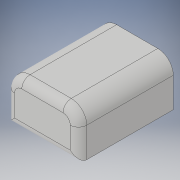
# Autodesk Inventor part: Aquamote3.2_housing_body_version2
Saved by Autodesk Inventor 2019 (Build 230136000, 136)
## iProperties
Created: 2018-04-22
Part Number: Aquamote3.2_housing_body_version2
Material: Generic
Document SubType Name: Modeling
Designer: Leon
Density: 1 g/cm^3
Appearance: Default
Author: Leon
Autodesk Inventor part; units mm, degrees
ref_plane "YZ Plane" through (0, 0, 0) normal (1, 0, 0) x (0, 1, 0)
ref_plane "XZ Plane" through (0, 0, 0) normal (0, 1, 0) x (-1, 0, 0)
ref_plane "XY Plane" through (0, 0, 0) normal (0, 0, 1) x (1, 0, 0)
sketch "Sketch1" plane through (0, 0, 0) normal (0, 0, 1) x (1, 0, 0)
  line L0 (0, 0) -> (35, 0)
  line L1 (35, 0) -> (35, 14.5)
  line L2 (27.5, 22) -> (7.5, 22)
  line L3 (0, 14.5) -> (0, 0)
  arc A0 (7.5, 22) -> (0, 14.5) centre (7.5, 14.5) ccw
  arc A1 (35, 14.5) -> (27.5, 22) centre (27.5, 14.5) ccw
  point P0 (35, 22)
  point P1 (0, 22)
  dimension "d0" = 35
  dimension "d1" = 22
  dimension "d2" = 7.5
  constraints: 8 end point, 4 point on circle, 4 point on line, 4 tangent, 2 centre point, 2 parallel, 1 equal radius, 1 horizontal, 1 perpendicular
  measures "d0" distance of point (0, 22) point (35, 22)
  measures "d1" distance of point (35, 22) L0.end
  measures "d2" radius of A0
extrude "Extrusion1" add sketch "Sketch1" along normal blind 46
sketch "Sketch2" plane through (0, 0, 0) normal (0, 0, -1) x (-1, 0, 0)
  line L0 (-9.5, 3) -> (-25.5, 3)
  line L1 (-29, 6.5) -> (-29, 15.5)
  line L2 (-25.5, 19) -> (-9.5, 19)
  line L3 (-6, 15.5) -> (-6, 14.8)
  arc A0 (-25.5, 19) -> (-29, 15.5) centre (-25.5, 15.5) ccw
  arc A1 (-29, 6.5) -> (-25.5, 3) centre (-25.5, 6.5) ccw
  arc A2 (-9.5, 3) -> (-6, 6.5) centre (-9.5, 6.5) ccw
  arc A3 (-6, 15.5) -> (-9.5, 19) centre (-9.5, 15.5) ccw
  line L4 (-29, 14.8) -> (-30.3, 14.8)
  line L5 (-30.3, 14.8) -> (-30.3, 13.2)
  line L6 (-30.3, 13.2) -> (-29, 13.2)
  line L7 (-29, 13.2) -> (-29, 14.8)
  line L8 (-6, 14.8) -> (-6, 13.2)
  line L9 (-6, 13.2) -> (-6, 6.5)
  line L10 (-6, 6.5) -> (-6, 15.5)
  line L11 (-6, 14.8) -> (-4.7, 14.8)
  line L12 (-4.7, 14.8) -> (-4.7, 13.2)
  line L13 (-4.7, 13.2) -> (-6, 13.2)
  point P0 (0, 0)
  point P1 (-29, 19)
  point P2 (-29, 3)
  point P3 (-6, 19)
  dimension "d5" = 23
  dimension "d6" = 16
  dimension "d7" = 3.5
  dimension "d8" = 6
  dimension "d9" = 19
  dimension "d80" = 1.3
  dimension "d81" = 1.6
  dimension "d82" = 4.2
  dimension "d88" = 1.3
  dimension "d89" = 1.6
  dimension "d90" = 4.2
  constraints: 28 end point, 13 tangent, 9 parallel, 8 point on circle, 6 point on line, 4 centre point, 3 equal radius, 2 horizontal, 2 perpendicular
  measures "d5" distance of point (-29, 19) point (-6, 19)
  measures "d6" distance of point (-29, 3) point (-29, 19)
  measures "d7" radius of A0
  measures "d8" distance from line of point (0, 0) L3
  measures "d9" distance from line of point (0, 0) L2
  measures "d80" distance of L6.end L5.end
  measures "d81" distance of L5.end L4.end
  measures "d82" distance between parallel lines of L2 L4
  measures "d88" distance between parallel lines of L12 L3
  measures "d89" distance between parallel lines of L11 L13
  measures "d90" distance between parallel lines of L11 L2
extrude "Extrusion2" cut sketch "Sketch2" against normal blind 43 contours L0 A1 L1 A0 L2 A3 L3 L8 L9 A2
chamfer "Chamfer1" distance 2 distance2 2.2 7 edges at (29, 11, 0) (27.9749, 17.9749, 0) (17.5, 19, 0) (7.0251, 17.9749, 0) (7.0251, 4.0251, 0) (17.5, 3, 0) (27.9749, 4.0251, 0) measured on face at (14.8333, 1, 0)
fillet "Fillet1" radius 2 7 edges at (29, 11, 43) (27.9749, 4.0251, 43) (17.5, 3, 43) (7.0251, 4.0251, 43) (7.0251, 17.9749, 43) (17.5, 19, 43) (27.9749, 17.9749, 43)
fillet "Fillet2" radius 4 6 edges at (17.5, 0, 46) (35, 7.25, 46) (32.8033, 19.8033, 46) (17.5, 22, 46) (2.1967, 19.8033, 46) (0, 7.25, 46)
sketch "Sketch4" plane through (0, 0, 0) normal (0, 0, -1) x (-1, 0, 0)
  circle A0 centre (-2, 11) radius 1.5
  line L0 (0, 14.5) -> (0, 0) projected
  line L1 (0, 0) -> (-35, 0) projected
  circle A1 centre (-33, 11) radius 1.5
  dimension "d20" = 3
  dimension "d21" = 2
  dimension "d22" = 11
  dimension "d23" = 3
  dimension "d24" = 11
  dimension "d25" = 31
  constraints: 2 centre point
  measures "d20" diameter of A0
  measures "d21" distance from line of L0 A0.centre
  measures "d22" distance from line of L1 A0.centre
  measures "d23" diameter of A1
  measures "d24" distance from line of L1 A1.centre
  measures "d25" distance of A0.centre A1.centre
hole "Hole1" at (2, 11, 0) direction (0, 0, 1) diameter 3 depth 15 tip angle 118
hole "Hole2" at (33, 11, 0) direction (0, 0, 1) diameter 3 depth 15 tip angle 118
thread "Thread1" size "M3x0.5" class "6H" standard "ANSI Metric M Profile" full length
thread "Thread2" size "M3x0.5" class "6H" standard "ANSI Metric M Profile" full length
sketch "Sketch6" plane through (33, 11, 0) normal (1, 0, 0) x (0, 1, 0)
  line L0 (1.5, 0) -> (1.5, 15)
  line L1 (1.5, 15) -> (1.1293, 15)
  line L2 (1.1293, 15) -> (1.1293, 0)
  line L3 (1.1293, 0) -> (1.5, 0)
  line L4 (0, -3) -> (0, 18) projected
  constraints: 8 end point
revolve "Revolution1" add sketch "Sketch6" angle 360 about axis through (33, 11, 0) along (0, 0, 1) separate body
sketch "Sketch5" plane through (33, 12.5, 0) normal (-1, 0, 0) x (0, 0, 1)
  line L0 (-0.2918, -0.0255) -> (-0.2501, -0.0255) construction
  line L1 (0.0416, -0.3456) -> (-0.0001, -0.4257) construction
  line L2 (-0.5001, -0.4257) -> (-0.5418, -0.3456) construction
  line L3 (-0.2084, -0.0255) -> (-0.2501, 0.0546) construction
  line L4 (-0.2501, 0.0546) -> (-0.2918, -0.0255) construction
  line L5 (-0.5001, -0.4257) -> (-0.4584, -0.3456) construction
  line L6 (-0.2084, -0.0255) -> (-0.0418, -0.3456)
  line L7 (-0.5418, -0.3456) -> (-0.4584, -0.3456) construction
  arc A0 (-0.5418, -0.3456) -> (-0.5001, -0.3709) centre (-0.5001, -0.3239) ccw construction
  line L8 (0.0416, -0.3456) -> (-0.0418, -0.3456) construction
  line L9 (-0.5001, -0.4257) -> (-0.5001, -0.3456) construction
  line L10 (-0.0001, -0.4257) -> (-0.0001, -0.3456) construction
  line L11 (-0.2501, 0.0546) -> (-0.2501, -0.0002) construction
  line L12 (-0.5001, -0.3709) -> (-0.0001, -0.3709)
  arc A1 (-0.5001, -0.3709) -> (-0.4584, -0.3456) centre (-0.5001, -0.3239) ccw
  line L13 (-0.0418, -0.3456) -> (-0.0001, -0.4257) construction
  line L14 (-0.4584, -0.3456) -> (-0.2918, -0.0255)
  line L15 (-0.0001, -0.0002) -> (-0.0001, 0.0177)
  line L16 (-0.0001, 0.0177) -> (-0.0001, -0.0002)
  line L17 (-0.0001, -0.0002) -> (0.0334, -0.0002)
  arc A2 (-0.0418, -0.3456) -> (-0.0001, -0.3709) centre (-0.0001, -0.3239) ccw
  arc A3 (-0.0001, -0.3709) -> (0.0416, -0.3456) centre (-0.0001, -0.3239) ccw construction
  arc A4 (-0.2501, -0.0002) -> (-0.2918, -0.0255) centre (-0.2501, -0.0471) ccw
  arc A5 (-0.2084, -0.0255) -> (-0.2501, -0.0002) centre (-0.2501, -0.0471) ccw
  line L18 (-0.2501, -0.0002) -> (-0.2501, -0.0255) construction
  line L19 (-0.2501, -0.0255) -> (-0.2084, -0.0255) construction
  dimension "d44" = 55
  dimension "d45" = 0.08
  dimension "d46" = 0.08
  dimension "Sketch5_ThreadOffset" = 0
  dimension "Sketch5_MajorRadius" = 0.3707
  dimension "d49" = 0.5
  dimension "Sketch5_MinorRadius" = 0
  constraints: 40 end point, 12 point on circle, 10 parallel, 8 tangent, 6 centre point, 6 collinear, 2 midpoint, 2 point on line, 1 horizontal, 1 perpendicular, 3 other
  measures "d44" angle of L6 L14
  measures "d45" distance of L3.end L0.end
  measures "d46" distance of L1.end L10.end
  measures "Sketch5_ThreadOffset" distance between parallel lines of L15 L10
  measures "Sketch5_MajorRadius" distance from line of L12 L15.start
  measures "d49" distance from line of L1.end L9
  measures "Sketch5_MinorRadius" distance edge to line of A5 L17
coil "Coil1" sketch "Sketch5" operation cut axis through (33, 11, 0) along (0, 0, 1) pitch 0.5005 turns 31.968032 hand right bodies 2
sketch "Sketch8" plane through (2, 11, 0) normal (1, 0, 0) x (0, 1, 0)
  line L0 (1.5, 0) -> (1.5, 15)
  line L1 (1.5, 15) -> (1.1293, 15)
  line L2 (1.1293, 15) -> (1.1293, 0)
  line L3 (1.1293, 0) -> (1.5, 0)
  line L4 (0, -3) -> (0, 18) projected
  constraints: 8 end point
revolve "Revolution2" add sketch "Sketch8" angle 360 about axis through (2, 11, 0) along (0, 0, 1) separate body
sketch "Sketch7" plane through (2, 12.5, 0) normal (-1, 0, 0) x (0, 0, 1)
  line L0 (-0.2918, -0.0255) -> (-0.2501, -0.0255) construction
  line L1 (0.0416, -0.3456) -> (-0.0001, -0.4257) construction
  line L2 (-0.5001, -0.4257) -> (-0.5418, -0.3456) construction
  line L3 (-0.2084, -0.0255) -> (-0.2501, 0.0546) construction
  line L4 (-0.2501, 0.0546) -> (-0.2918, -0.0255) construction
  line L5 (-0.5001, -0.4257) -> (-0.4584, -0.3456) construction
  line L6 (-0.2084, -0.0255) -> (-0.0418, -0.3456)
  line L7 (-0.5418, -0.3456) -> (-0.4584, -0.3456) construction
  arc A0 (-0.5418, -0.3456) -> (-0.5001, -0.3709) centre (-0.5001, -0.3239) ccw construction
  line L8 (0.0416, -0.3456) -> (-0.0418, -0.3456) construction
  line L9 (-0.5001, -0.4257) -> (-0.5001, -0.3456) construction
  line L10 (-0.0001, -0.4257) -> (-0.0001, -0.3456) construction
  line L11 (-0.2501, 0.0546) -> (-0.2501, -0.0002) construction
  line L12 (-0.5001, -0.3709) -> (-0.0001, -0.3709)
  arc A1 (-0.5001, -0.3709) -> (-0.4584, -0.3456) centre (-0.5001, -0.3239) ccw
  line L13 (-0.0418, -0.3456) -> (-0.0001, -0.4257) construction
  line L14 (-0.4584, -0.3456) -> (-0.2918, -0.0255)
  line L15 (-0.0001, -0.0002) -> (-0.0001, 0.0177)
  line L16 (-0.0001, 0.0177) -> (-0.0001, -0.0002)
  line L17 (-0.0001, -0.0002) -> (0.0334, -0.0002)
  arc A2 (-0.0418, -0.3456) -> (-0.0001, -0.3709) centre (-0.0001, -0.3239) ccw
  arc A3 (-0.0001, -0.3709) -> (0.0416, -0.3456) centre (-0.0001, -0.3239) ccw construction
  arc A4 (-0.2501, -0.0002) -> (-0.2918, -0.0255) centre (-0.2501, -0.0471) ccw
  arc A5 (-0.2084, -0.0255) -> (-0.2501, -0.0002) centre (-0.2501, -0.0471) ccw
  line L18 (-0.2501, -0.0002) -> (-0.2501, -0.0255) construction
  line L19 (-0.2501, -0.0255) -> (-0.2084, -0.0255) construction
  dimension "d62" = 55
  dimension "d63" = 0.08
  dimension "d64" = 0.08
  dimension "Sketch7_ThreadOffset" = 0
  dimension "Sketch7_MajorRadius" = 0.3707
  dimension "d67" = 0.5
  dimension "Sketch7_MinorRadius" = 0
  constraints: 40 end point, 12 point on circle, 10 parallel, 8 tangent, 6 centre point, 6 collinear, 2 midpoint, 2 point on line, 1 horizontal, 1 perpendicular, 3 other
  measures "d62" angle of L6 L14
  measures "d63" distance of L3.end L0.end
  measures "d64" distance of L1.end L10.end
  measures "Sketch7_ThreadOffset" distance between parallel lines of L15 L10
  measures "Sketch7_MajorRadius" distance from line of L12 L15.start
  measures "d67" distance from line of L1.end L9
  measures "Sketch7_MinorRadius" distance edge to line of A5 L17
coil "Coil2" sketch "Sketch7" operation cut axis through (2, 11, 0) along (0, 0, 1) pitch 0.5005 turns 31.968032 hand right bodies 3
extrude "Extrusion3" cut sketch "Sketch2" against normal blind 42 contours L6 L5 L4 L1 bodies 1
extrude "Extrusion4" cut sketch "Sketch2" against normal blind 42 contours L8 L11 L12 L13 bodies 1
equation "\"d44\" = d51"
equation "\"d45\" = 0.160083 * Sketch5_Pitch"
equation "\"d46\" = 0.160083 * Sketch5_Pitch"
equation "\"d49\" = Sketch5_Pitch"
equation "\"d62\" = d69"
equation "\"d63\" = 0.160083 * Sketch7_Pitch"
equation "\"d64\" = 0.160083 * Sketch7_Pitch"
equation "\"d67\" = Sketch7_Pitch"
equation "\"d51\" = 55deg"
equation "\"Sketch5_Pitch\" = 0.5"
equation "\"d69\" = 55deg"
equation "\"Sketch7_Pitch\" = 0.5"
body "Solid1"
body "Solid2"
body "Solid3"
